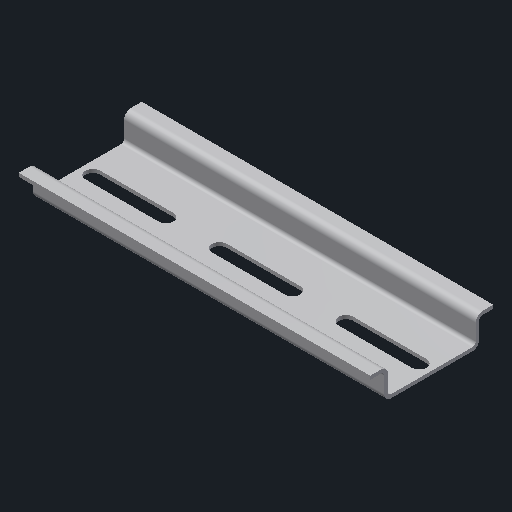
# Autodesk Inventor part: DIN Rail (TS) 35mm Wide v1-01
Saved by Autodesk Inventor 2025.2 (Build 292293000, 293)
## iProperties
Created: 2016-05-16
Part Number: DIN Rail (TS) 35mm Wide v1-01
Material: Steel
Document SubType Name: Sheet Metal
Designer: Neil Holmes
Mass: 34.3036 g
Surface Area: 92.0243 cm^2
Volume: 4.36989 cm^3
Density: 7.85 g/cm^3
Sheet Metal Rule: 1.0mm Mild Steel
Appearance: Steel BZP
Author: Neil Holmes
Autodesk Inventor part; units mm, degrees
ref_plane "YZ Plane" through (0, 0, 0) normal (1, 0, 0) x (0, 1, 0)
ref_plane "XZ Plane" through (0, 0, 0) normal (0, 1, 0) x (-1, 0, 0)
ref_plane "XY Plane" through (0, 0, 0) normal (0, 0, 1) x (1, 0, 0)
sketch "Base Pattern" plane through (0, 0, 0) normal (0, 1, 0) x (-1, 0, 0)
  line L0 (50, 13.5) -> (-50, 13.5)
  line L1 (-50, 13.5) -> (-50, -13.5)
  line L2 (-50, -13.5) -> (50, -13.5)
  line L3 (50, -13.5) -> (50, 13.5)
  line L4 (50, 13.5) -> (-50, -13.5) construction
  line L5 (-50, 13.5) -> (50, -13.5) construction
  point P0 (0, 0)
  dimension "Length" = 100
  dimension "Base_Width" = 27
  constraints: 12 end point, 2 midpoint, 2 parallel, 1 horizontal, 1 perpendicular
  measures "Length" distance of L2.end L1.end
  measures "Base_Width" distance of L1.end L0.end
sketch "Slot Pattern Set-Out" plane through (0, 0, 0) normal (0, 1, 0) x (-1, 0, 0)
  line L0 (0, -25) -> (0, 25)
  line L1 (10.385, 2.115) -> (-10.385, 2.115)
  line L2 (-10.385, -2.115) -> (10.385, -2.115)
  arc A0 (10.385, -2.115) -> (10.385, 2.115) centre (10.385, 0) ccw
  arc A1 (-10.385, 2.115) -> (-10.385, -2.115) centre (-10.385, 0) ccw
  line L3 (32, 0) -> (-32, 0) construction
  line L4 (10.385, 0) -> (-10.385, 0) construction
  point P0 (0, 0)
  point P1 (0, 0)
  point P2 (0, 0)
  point P3 (0, 0)
  dimension "Slot_Length" = 20.77
  dimension "Slot_Dia" = 4.23
  dimension "Pattern_Length" = 64
  constraints: 10 end point, 6 coincident, 4 point on circle, 4 tangent, 3 midpoint, 2 centre point, 2 horizontal, 1 parallel, 1 vertical
  measures "Slot_Length" distance of L4.start L4.end
  measures "Slot_Dia" diameter of A1
  measures "Pattern_Length" distance of L3.start L3.end
extrude "Plate1" add sketch "Base Pattern" along normal blind 1
sketch "Sketch3" plane through (-50, 0, -12.5) normal (0, 0, -1) x (-1, 0, 0)
  line L0 (-100, 0) -> (0, 0)
  line L1 (0, 0) -> (0, 7.5)
  line L2 (0, 7.5) -> (-100, 7.5)
  line L3 (-100, 7.5) -> (-100, 0)
  constraints: 4 end point, 4 other
edge flange "Flange Side" height 7.5 angle 90 thickness 1 bend radius 1 thickness toward (0, 0, -1) relief tear relief width 1 relief depth 0.5 corner gap 1 corner form 0 edges at (0, 1, -13.5) (0, 1, 13.5) wall of the first edge with corners at (50, 0, -12.5) (-50, 0, -12.5) (-50, 7.5, -12.5) (50, 7.5, -12.5)
bend "Bend1"
corner "Corner1"
sketch "Sketch4" plane through (-50, 7.5, 13.5) normal (0, 1, 0) x (-1, 0, 0)
  line L0 (-100, 0) -> (0, 0)
  line L1 (0, 0) -> (0, 4)
  line L2 (0, 4) -> (-100, 4)
  line L3 (-100, 4) -> (-100, 0)
  constraints: 4 end point, 4 other
edge flange "Flange Nib" height 5 angle 90 thickness 1 bend radius 1 thickness toward (0, 1, 0) relief tear relief width 1 relief depth 0.5 corner gap 1 corner form 0 edges at (0, 7.5, 13.5) (0, 7.5, -13.5) wall of the first edge with corners at (50, 7.5, 13.5) (-50, 7.5, 13.5) (-50, 7.5, 17.5) (50, 7.5, 17.5)
bend "Bend2"
corner "Corner2"
extrude "Slot Cut-Out" cut sketch "Slot Pattern Set-Out" along normal blind 1
pattern_linear "Slot Pattern" count 2 spacing 36 along (1, 0, 0) of "Slot Cut-Out"
mirror "Slot Patern Mirror" about plane through (0, 0, 0) normal (1, 0, 0) of "Slot Cut-Out", "Slot Pattern"
equation "\"Slot_Length\" = Slot_Length_Effective"
equation "\"d28\" = Thickness"
equation "\"d30\" = 0.6 * Slots_Integer"
equation "\"d32\" = Slot_Spacing"
equation "\"d33\" = Thickness"
equation "\"d8\" = BendReliefWidth"
equation "\"d9\" = BendReliefDepth"
equation "\"d10\" = MinimumRemnant"
equation "\"d11\" = BendRadius"
equation "\"d12\" = Flange_Height"
equation "\"d14\" = BendRadius"
equation "\"d15\" = CornerReliefSize"
equation "\"d16\" = GapSize"
equation "\"d17\" = JacobiRadiusSize"
equation "\"d18\" = BendReliefWidth"
equation "\"d19\" = BendReliefDepth"
equation "\"d20\" = MinimumRemnant"
equation "\"d21\" = BendRadius"
equation "\"d22\" = Flange_Nib"
equation "\"d24\" = BendRadius"
equation "\"d25\" = CornerReliefSize"
equation "\"d26\" = GapSize"
equation "\"d27\" = JacobiRadiusSize"
equation "\"BendRadius\" = Thickness"
equation "\"BendReliefWidth\" = Thickness"
equation "\"BendReliefDepth\" = 0.5 * Thickness"
equation "\"CornerReliefSize\" = 4 * Thickness"
equation "\"MinimumRemnant\" = 2 * Thickness"
equation "\"TransitionRadius\" = BendRadius"
equation "\"JacobiRadiusSize\" = BendRadius"
equation "\"GapSize\" = Thickness"
equation "\"Flange_Height\" = 7.5"
equation "\"Slot_Spacing\" = 36"
equation "\"Flange_Nib\" = 5"
equation "\"Slot_Length_Tab\" = 25"
equation "\"Slot_Length_Effective\" = Slot_Length_Tab - Slot_Dia"
equation "\"Thickness\" = 1"
equation "\"Slots_Integer\" = 2.777778"
body "Solid1"
